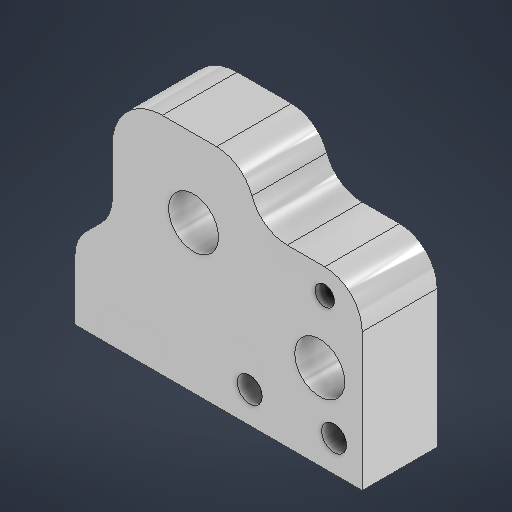
# Autodesk Inventor part: Lagerblock Dribbler
Saved by Autodesk Inventor 2025.2 (Build 292293000, 293)
## iProperties
Created: 2024-11-14
Part Number: Lagerblock Dribbler
Material: Generisch
Document SubType Name: Modeling
Designer: Fabian
Density: 1 g/cm^3
Appearance: Aluminium - poliert
Author: Fabian
Autodesk Inventor part; units mm, degrees
note: some values were not read from the file. Chosen so that the rebuilt part matches the saved one: direction of "Bohrung5".
ref_plane "YZ Plane" through (0, 0, 0) normal (1, 0, 0) x (0, 1, 0)
ref_plane "XZ Plane" through (0, 0, 0) normal (0, 1, 0) x (-1, 0, 0)
ref_plane "XY Plane" through (0, 0, 0) normal (0, 0, 1) x (1, 0, 0)
sketch "Skizze2" plane through (0, 0, 0) normal (0, 0, 1) x (1, 0, 0)
  line L0 (0, 0) -> (23, 0)
  line L1 (23, 0) -> (23, 18)
  line L2 (23, 18) -> (3, 18)
  line L3 (0, 6) -> (0, 0)
  line L4 (0, 0) -> (0, 6)
  line L5 (0, 6) -> (3, 6)
  line L6 (3, 6) -> (3, 18)
  line L7 (0, 6) -> (3, 9)
  line L8 (0, 0) -> (19.6, 0)
  line L9 (19.6, 0) -> (19.6, 6.8)
  line L10 (23, 0) -> (23, 12)
  line L11 (9.5, 0) -> (9.5, 11.8)
  line L12 (14, 14) -> (23, 14)
  line L13 (14, 14) -> (14, 18)
  dimension "d21" = 18
  dimension "d22" = 6
  dimension "d23" = 3
  dimension "d24" = 23
  dimension "d25" = 45
  dimension "d26" = 19.6
  dimension "d27" = 6.8
  dimension "d28" = 12
  dimension "d30" = 11.8
  dimension "d31" = 9.5
  dimension "d36" = 14
  dimension "d37" = 9
  constraints: 28 end point, 6 point on line, 5 perpendicular, 2 coincident, 2 parallel, 1 horizontal, 1 vertical
  measures "d21" distance of L1.end L0.end
  measures "d22" distance of L3.start L0.start
  measures "d23" distance of L3.start L5.end
  measures "d24" distance of L0.start L0.end
  measures "d25" angle of L5 L7
  measures "d26" distance of L0.start L8.end
  measures "d27" distance of L8.end L9.end
  measures "d28" distance of L0.end L10.end
  measures "d30" distance of L11.start L11.end
  measures "d31" distance between parallel lines of L3 L11
  measures "d36" distance between parallel lines of L8 L12
  measures "d37" distance between parallel lines of L1 L13
extrude "Extrusion1" add sketch "Skizze2" along normal mid plane 6 contours L3 L5 L6 L2 L13 L12 L1 L0 | L7 L6 L5
hole "Bohrung1" at (19.6, 6.8, 0) at (9.5, 11.8, 0) direction (0, 0, -1) diameter 4 end through all both
fillet "Rundung1" radius 3 4 edges at (0, 6, 0) (3, 9, 0) (23, 14, 0) (14, 14, 0)
fillet "Rundung2" radius 4 1 edges at (3, 18, 0)
fillet "Rundung3" radius 3 1 edges at (14, 18, 0)
sketch "Skizze3" plane through (0, 0, 3) normal (0, -1, 0) x (1, 0, 0)
  line L0 (0, -3) -> (3.5, -3) construction
  line L1 (3.5, -3) -> (10.5, -3) construction
  line L2 (10.5, -3) -> (17.5, -3) construction
  dimension "d50" = 3.5
  dimension "d51" = 7
  dimension "d52" = 7
  constraints: 6 end point, 3 coincident, 2 point on line, 1 horizontal
  measures "d50" distance of L0.start L0.end
  measures "d51" distance of L0.end L1.end
  measures "d52" distance of L1.end L2.end
hole "Bohrung2" at (3.5, 0, 0) at (10.5, 0, 0) direction (0, 1, 0) diameter 2.459 depth 7 tip angle 118 thread size "M3x0.5" class "6H" standard "ISO Metric profile"
hole "Bohrung3" at (17.5, 0, 0) direction (0, 1, 0) diameter 2.459 depth 4 tip angle 118 thread size "M3x0.5" class "6H" standard "ISO Metric profile"
sketch "Skizze4" plane through (0, 0, 3) normal (0, 0, 1) x (1, 0, 0)
  line L0 (14, 0) -> (14, 2.5)
  line L1 (20.75, 0) -> (20.75, 2.5)
  line L2 (0, 4.7574) -> (0, 0) projected
  line L3 (0, 0) -> (0, 4.7574)
  point P0 (23, 0)
  dimension "d71" = 2.5
  dimension "d72" = 2.5
  dimension "d89" = 14
  dimension "d90" = 6.75
  constraints: 6 end point, 3 vertical, 2 coincident
  measures "d71" distance of L0.start L0.end
  measures "d72" distance of L1.start L1.end
  measures "d89" distance between parallel lines of L2 L0
  measures "d90" distance between parallel lines of L1 L0
hole "Bohrung4" at (14, 2.5, 3) at (20.75, 2.5, 3) direction (0, 0, -1) diameter 2 end through all
sketch "Skizze5" plane through (0, 0, 3) normal (0, 0, 1) x (1, 0, 0)
  line L0 (20, 0) -> (20, 12)
  line L1 (0, 4.7574) -> (0, 0) projected
  line L2 (0, 0) -> (0, 4.7574)
  dimension "d81" = 12
  dimension "d91" = 20
  constraints: 4 end point, 1 coincident, 1 vertical
  measures "d81" distance of L0.start L0.end
  measures "d91" distance between parallel lines of L1 L0
hole "Bohrung5" at (20, 12, 3) direction (0, 0, -1) diameter 1.567 depth 6 thread size "M2x0.4" class "6H" standard "ISO Metric profile"
